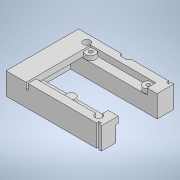
# Autodesk Inventor part: Стойка под электроннику
Saved by Autodesk Inventor 2020 (Build 240168000, 168)
## iProperties
Created: 2021-04-05
Part Number: Стойка под электроннику
Material: Типовые
Document SubType Name: Обычные детали
Designer: Антон
Density: 1 g/cm^3
Appearance: По умолчанию
Author: Антон
Autodesk Inventor part; units mm, degrees
ref_plane "YZ Plane" through (0, 0, 0) normal (1, 0, 0) x (0, 1, 0)
ref_plane "XZ Plane" through (0, 0, 0) normal (0, 1, 0) x (-1, 0, 0)
ref_plane "XY Plane" through (0, 0, 0) normal (0, 0, 1) x (1, 0, 0)
sketch "Эскиз1" plane through (0, 0, 0) normal (0, 1, 0) x (-1, 0, 0)
  line L0 (0, 0) -> (76, 0)
  line L1 (76, 0) -> (76, -57.8)
  line L2 (76, -57.8) -> (0, -57.8)
  line L3 (0, -57.8) -> (0, 0)
  line L4 (0, -28.9) -> (34.5, -28.9)
  line L5 (69, -13.4) -> (0, -13.4)
  line L6 (0, -13.4) -> (0, -44.4)
  line L7 (0, -44.4) -> (69, -44.4)
  line L8 (69, -44.4) -> (69, -13.4)
  line L9 (69, -13.4) -> (0, -44.4) construction
  line L10 (0, -13.4) -> (69, -44.4) construction
  line L11 (0, -13.4) -> (4, -13.4)
  point P0 (0, -13.4)
  dimension "d0" = 76
  dimension "d1" = 57.8
  dimension "d3" = 31
  dimension "d4" = 69
  constraints: 24 end point, 4 horizontal, 4 parallel, 3 midpoint, 2 perpendicular, 1 point on line
  measures "d0" distance of L1.end L2.end
  measures "d1" distance of L0.end L1.end
  measures "d3" distance of L6.end L5.end
  measures "d4" distance of L6.end L7.end
extrude "Выдавливание1" add sketch "Эскиз1" along normal blind 17.5 contours L0 L1 L2 L3 L7 L8 L5
sketch "Эскиз2" plane through (0, 17.5, 0) normal (0, 1, 0) x (1, 0, 0)
  line L0 (0, 0) -> (0, 6.4)
  line L1 (0, 0) -> (0, 57.8) projected
  line L2 (0, 6.4) -> (-8, 6.4)
  line L3 (-8, 6.4) -> (-60, 6.4)
  line L4 (-60, 6.4) -> (-60, 51.4)
  line L5 (-60, 51.4) -> (-8, 51.4)
  line L6 (-8, 51.4) -> (-8, 6.4)
  line L7 (-76, 57.8) -> (-76, 0) projected
  line L8 (-76, 0) -> (0, 0) projected
  point P0 (-60, 22)
  dimension "d9" = 6.4
  dimension "d10" = 8
  dimension "d11" = 52
  dimension "d12" = 45
  dimension "d16" = 57.8
  dimension "d17" = 76
  constraints: 12 end point, 2 parallel, 2 perpendicular, 2 point on line, 1 horizontal
  measures "d9" distance of L0.start L0.end
  measures "d10" distance of L0.end L2.end
  measures "d11" distance of L4.end L5.end
  measures "d12" distance of L3.end L4.end
  measures "d16" distance of L7.start L7.end
  measures "d17" distance of L7.end L0.start
extrude "Выдавливание2" cut sketch "Эскиз2" against normal blind 5
sketch "Эскиз29" plane through (-69, 0, -13.4) normal (1, 0, 0) x (0, 0, -1)
  line L0 (0, 17.5) -> (0, 12.5) projected
  line L1 (31, 12.5) -> (31, 17.5) projected
  line L2 (0, 17.5) -> (31, 17.5) projected
  line L3 (0, 12.5) -> (31, 12.5)
  point P0 (-13.4, 0)
  constraints: 2 end point, 1 perpendicular
extrude "Выдавливание23" add sketch "Эскиз29" along normal up to surface (9 mm away)
sketch "Эскиз3" plane through (0, 12.5, 0) normal (0, 1, 0) x (1, 0, 0)
  line L0 (-8, 6.4) -> (-60, 6.4) projected
  line L1 (-8, 51.4) -> (-8, 6.4) projected
  line L2 (-8, 51.4) -> (-11, 51.4)
  line L3 (-60, 51.4) -> (-8, 51.4) projected
  line L4 (-11, 51.4) -> (-11, 48.4)
  circle A0 centre (-11, 48.4) radius 4
  line L5 (-8, 6.4) -> (-60, 6.4) projected
  line L6 (-60, 51.4) -> (-8, 51.4) projected
  line L7 (-60, 51.4) -> (-57, 51.4)
  line L8 (-57, 51.4) -> (-57, 48.4)
  circle A1 centre (-57, 48.4) radius 4
  line L9 (-34, 6.4) -> (-34, 9.9)
  circle A2 centre (-34, 9.9) radius 3.5
  point P0 (-74.9, 17.65)
  point P1 (-74.9, 50.35)
  point P2 (-8, 44.4)
  point P3 (-8.3542, 51.4)
  point P4 (-8, 51.0458)
  point P5 (-59.6458, 51.4)
  point P6 (-54.3542, 51.4)
  dimension "d35" = 3
  dimension "d36" = 3
  dimension "d37" = 8
  dimension "d205" = 3
  dimension "d206" = 3
  dimension "d207" = 8
  dimension "d214" = 3.5
  dimension "d215" = 7
  constraints: 10 end point, 3 centre point, 3 coincident, 2 point on line, 2 vertical, 1 midpoint, 1 perpendicular
  measures "d35" distance of L1.start L2.end
  measures "d36" distance of L2.end L4.end
  measures "d37" diameter of A0
  measures "d205" distance of L3.start L7.end
  measures "d206" distance of L7.end L8.end
  measures "d207" diameter of A1
  measures "d214" distance of L9.start L9.end
  measures "d215" diameter of A2
extrude "Выдавливание5" add sketch "Эскиз3" along normal blind 3.5 contours L1 A0 L2 | A0 L1 | L1 A0 L3 L2 | L2 L3 A0 | L3 A1 | A2 picked at (-57.1322, 46.7573)
sketch "Эскиз4" plane through (-71.3, 16, -19.65) normal (0, 1, 0) x (0, 0, -1)
  arc A0 (31.75, -57.6542) -> (26.1042, -63.3) centre (28.75, -60.3) ccw projected
  line L0 (26.1042, -11.3) -> (31.3958, -11.3) projected
  arc A1 (26.1042, -11.3) -> (31.75, -16.9458) centre (28.75, -14.3) ccw projected
  line L1 (31.75, -11.6542) -> (31.75, -16.9458) projected
  arc A2 (31.75, -11.6542) -> (31.3958, -11.3) centre (28.75, -14.3) ccw projected
  point P0 (31.75, -57.1028)
  constraints: 2 coincident
hole "Отверстие1" at (-11, 16, -48.4) at (-57, 16, -48.4) direction (0, -1, 0) diameter 3 depth 5
sketch "Эскиз5" plane through (0, 12.5, 0) normal (0, 1, 0) x (1, 0, 0)
  line L0 (-60, 51.4) -> (-8, 51.4) projected
  line L1 (-8, 6.4) -> (-8.2, 6.4)
  line L2 (-8.2, 6.4) -> (-8.2, 6.05)
  line L3 (-8, 6.4) -> (-60, 6.4) projected
  line L4 (-60, 51.4) -> (-63.4, 51.4)
  line L5 (-63.4, 51.4) -> (-63.4, 51.75)
  line L6 (-8, 51.4) -> (-8, 6.4) projected
  point P0 (-21.2, 2.05)
  point P1 (-57.2, 6.4)
  point P2 (-8, 44.4)
  point P3 (-20.7569, 6.4)
  point P4 (-60, 6.4)
  dimension "d196" = 0.35
  dimension "d200" = 0.35
  dimension "d208" = 3.4
  dimension "d209" = 0.2
  constraints: 8 end point, 2 perpendicular, 1 horizontal, 1 point on line, 1 other
  measures "d196" distance of L4.end L5.end
  measures "d200" distance of L1.end L2.end
  measures "d208" distance of L0.start L4.end
  measures "d209" distance of L1.start L1.end
hole "Отверстие2" at (-63.4, 12.5, -51.75) at (-8.2, 12.5, -6.05) direction (0, -1, 0) diameter 3.2 end through all countersink diameter 5.8 countersink angle 90
sketch "Эскиз27" plane through (0, 12.5, 0) normal (0, 1, 0) x (1, 0, 0)
  arc A0 (-53.0282, 48.8739) -> (-50.5212, 51.4) centre (-53.4, 51.75) ccw projected
  circle A1 centre (-63.4, 51.75) radius 2.9 projected
  circle A2 centre (-63.4, 51.75) radius 1.6 projected
  circle A3 centre (-8.2, 6.05) radius 1.6 projected
  arc A4 (-11.0788, 6.4) -> (-8, 8.9431) centre (-8.2, 6.05) ccw projected
  line L0 (-8, 8.9431) -> (-8, 6.4) projected
  line L1 (-8, 6.4) -> (-11.0788, 6.4) projected
  line L2 (-8, 6.4) -> (-60, 6.4) projected
  line L3 (-34, 6.4) -> (-34, 10.4)
  point P0 (0, 0)
  point P1 (-65, 49.3313)
  point P2 (-50.5212, 51.4)
  dimension "d213" = 4
  constraints: 2 end point, 1 midpoint, 1 vertical
  measures "d213" distance of L3.start L3.end
extrude "Выдавливание21" cut sketch "Эскиз27" along normal up to surface (5 mm away) contours A1 | A2 | A3 L1 L0 | A3 L0 A4 L1 picked at (-8.6134, 5.2227)
sketch "Эскиз10" plane through (0, 0, 0) normal (0, -1, 0) x (1, 0, 0)
  line L0 (0, 0) -> (0, -13.4) projected
  line L1 (0, -13.4) -> (-4, -13.4)
  line L2 (-4, -13.4) -> (-4, -11.4)
  line L3 (-4, -11.4) -> (0, -11.4)
  line L4 (0, -11.4) -> (0, -13.4)
  dimension "d109" = 4
  dimension "d110" = 2
  constraints: 8 end point, 2 parallel, 1 horizontal, 1 perpendicular
  measures "d109" distance of L2.end L3.end
  measures "d110" distance of L1.end L2.end
extrude "Выдавливание9" cut sketch "Эскиз10" against normal up to surface (12.5 mm away)
sketch "Эскиз11" plane through (-76, 0, 0) normal (0, 0, 1) x (1, 0, 0)
  line L0 (76, 0) -> (76, 17.5) projected
  line L1 (76, 0) -> (76, 0)
  line L2 (76, 17.5) -> (76, 17.5)
  line L3 (76, 0) -> (74, 0)
  line L4 (76, 17.5) -> (74, 17.5)
  line L5 (74, 0) -> (72, 0)
  line L6 (72, 0) -> (72, 17.5)
  line L7 (72, 17.5) -> (74, 17.5)
  line L8 (74, 17.5) -> (74, 0)
  line L9 (0, 17.5) -> (76, 17.5) projected
  dimension "d113" = 2
  dimension "d115" = 2
  constraints: 16 end point, 3 horizontal, 2 equal length, 2 parallel, 2 point on line, 1 collinear, 1 perpendicular
  measures "d113" distance of L1.end L3.end
  measures "d115" distance between parallel lines of L8 L6
extrude "Выдавливание10" cut sketch "Эскиз11" against normal blind 2 contours L5 L6 L7 L8
ref_plane "РабПлоскость2" through (-76, 0, -28.9) normal (0, 0, 1) x (1, 0, 0)
mirror "Зеркальное отражение1" about plane through (-76, 0, -28.9) normal (0, 0, 1) of "Выдавливание10"
sketch "Эскиз12" plane through (0, 0, 0) normal (0, -1, 0) x (1, 0, 0)
  line L0 (-36, -57.8) -> (-40, -57.8) construction
  line L1 (0, -57.8) -> (-76, -57.8) projected
  line L2 (-36, -55.75) -> (-40, -55.75)
  line L3 (-40, -59.85) -> (-36, -59.85)
  arc A0 (-36, -59.85) -> (-36, -55.75) centre (-36, -57.8) ccw
  arc A1 (-40, -55.75) -> (-40, -59.85) centre (-40, -57.8) ccw
  line L4 (-60, -51.4) -> (-60, -6.4) projected
  line L5 (-60, -51.4) -> (-8, -51.4) projected
  line L6 (-8, -51.4) -> (-8, -44.4) projected
  line L7 (-8, -44.4) -> (0, -44.4) projected
  line L8 (0, -44.4) -> (0, -57.8) projected
  line L9 (0, -57.8) -> (-2, -57.8) projected
  line L10 (-76, -57.8) -> (-76, 0) projected
  line L11 (-76, 0) -> (-4, 0) projected
  line L12 (0, 0) -> (0, -13.4) projected
  line L13 (0, -13.4) -> (-8, -13.4) projected
  line L14 (-8, -13.4) -> (-8, -8.9431) projected
  line L15 (-11.0788, -6.4) -> (-60, -6.4) projected
  line L16 (-36, -55.75) -> (-40, -55.75)
  line L17 (-2, -57.8) -> (-2, -55.8) projected
  line L18 (-2, -55.8) -> (-4, -55.8) projected
  line L19 (-4, -55.8) -> (-4, -57.8) projected
  line L20 (-4, -57.8) -> (-76, -57.8) projected
  line L21 (-4, 0) -> (-4, -2) projected
  line L22 (-4, -2) -> (-2, -2) projected
  line L23 (-2, -2) -> (-2, 0) projected
  line L24 (-2, 0) -> (0, 0) projected
  circle A2 centre (-63.4, -51.75) radius 2.9 projected
  arc A3 (-8, -8.9431) -> (-11.0788, -6.4) centre (-8.2, -6.05) ccw projected
  point P0 (-38, -57.8)
  point P1 (-41, -51.4)
  point P2 (-35, -51.4)
  point P3 (-42.05, -57.8)
  point P4 (-33.95, -57.8)
  point P5 (-35, -51.4)
  point P6 (-42.05, -57.8)
  point P7 (-33.95, -57.8)
  point P8 (-4, -57.8)
  point P9 (-2, -57.8)
  dimension "d118" = 2
  dimension "d210" = 2.05
  constraints: 10 end point, 4 point on circle, 4 tangent, 2 centre point, 2 midpoint, 1 horizontal, 1 parallel, 1 point on line
  measures "d118" distance of point (-38, -57.8) L0.end
  measures "d210" radius of A1
extrude "Выдавливание11" cut sketch "Эскиз12" against normal through all contours L1 L19 L18 L17 | A0 L3 A1 L1 | L1 A1 L2 A0
sketch "Эскиз14" plane through (0, 17.5, 0) normal (0, 1, 0) x (1, 0, 0)
  line L0 (-60, 51.4) -> (-8, 51.4) projected
  line L1 (-38, 51.4) -> (-38, 53.0067)
  line L2 (0, 57.8) -> (-2, 57.8) projected
  line L3 (-32.95, 57.8) -> (-30.95, 57.8)
  line L4 (-30.95, 57.8) -> (-30.95, 49.4)
  line L5 (-30.95, 49.4) -> (-32.95, 49.4)
  line L6 (-32.95, 49.4) -> (-32.95, 57.8)
  line L7 (-30.95, 49.4) -> (-45.05, 49.4)
  line L8 (-45.05, 49.4) -> (-45.05, 51.4)
  line L9 (-45.05, 51.4) -> (-30.95, 51.4)
  line L10 (-30.95, 51.4) -> (-30.95, 49.4)
  line L11 (-45.05, 49.4) -> (-43.05, 49.4)
  line L12 (-43.05, 49.4) -> (-43.05, 57.8)
  line L13 (-43.05, 57.8) -> (-45.05, 57.8)
  line L14 (-45.05, 57.8) -> (-45.05, 49.4)
  line L15 (-60, 51.4) -> (-8, 51.4) projected
  line L16 (-40, 55.75) -> (-36, 55.75) projected
  line L17 (-41, 51.4) -> (-34.5, 51.4) projected
  line L18 (-36, 55.75) -> (-40, 55.75) projected
  line L19 (-4, 57.8) -> (-33.95, 57.8) projected
  line L20 (-42.05, 57.8) -> (-76, 57.8) projected
  point P0 (0, 0)
  point P1 (-28.95, 57.8)
  point P2 (-32.95, 51.4)
  point P3 (-47.05, 54.4893)
  point P4 (-49.4, 51.4)
  point P5 (-43.05, 51.4)
  point P6 (-34.5, 51.4)
  point P7 (-30.95, 51.4)
  point P8 (-34.5, 51.4)
  point P9 (-38, 55.75)
  dimension "d136" = 2
  dimension "d137" = 2
  dimension "d211" = 1
  dimension "d212" = 1
  constraints: 26 end point, 6 parallel, 4 collinear, 3 horizontal, 3 perpendicular, 2 midpoint, 2 point on line, 1 vertical, 1 other
  measures "d136" distance between parallel lines of L6 L4
  measures "d137" distance between parallel lines of L9 L7
  measures "d211" distance from line of L6 L19.end
  measures "d212" distance from line of L12 L20.start
ref_plane "РабПлоскость4" through (0, 8.75, 0) normal (0, 1, 0) x (1, 0, 0)
extrude "Выдавливание12" cut sketch "Эскиз14" against normal mid plane 5 from surface at -8.75
chamfer "Фаска5" distance 1 angle 45 4 edges at (-32.95, 8.75, -51.4) (-43.05, 8.75, -51.4) (-45.05, 8.75, -49.4) (-30.95, 8.75, -49.4)
sketch "Эскиз21" plane through (0, 0, 0) normal (0, -1, 0) x (1, 0, 0)
  line L0 (-74, -2.7) -> (-49, -2.7)
  line L1 (-49, -2.7) -> (-49, -10.7)
  line L2 (-49, -10.7) -> (-74, -10.7)
  line L3 (-74, -10.7) -> (-74, -2.7)
  line L4 (-76, 0) -> (-4, 0) projected
  line L5 (-76, -57.8) -> (-76, 0) projected
  point P0 (0, 0)
  dimension "d167" = 8
  dimension "d168" = 25
  dimension "d169" = 2.7
  dimension "d170" = 2
  constraints: 8 end point, 2 parallel, 1 horizontal, 1 perpendicular
  measures "d167" distance of L0.end L1.end
  measures "d168" distance of L1.end L2.end
  measures "d169" distance between parallel lines of L4 L0
  measures "d170" distance between parallel lines of L5 L3
extrude "Выдавливание17" cut sketch "Эскиз21" against normal blind 13.5
sketch "Эскиз22" plane through (-76, 0, -57.8) normal (-1, 0, 0) x (0, 0, 1)
  line L0 (47.1, 0) -> (55.1, 0) projected
  line L1 (47.1, 0) -> (47.1, 13.5) projected
  line L2 (47.1, 13.5) -> (55.1, 13.5) projected
  line L3 (55.1, 0) -> (55.1, 13.5) projected
  line L4 (47.1, 0) -> (47.1, 13.5) projected
  line L5 (47.1, 6.75) -> (55.1, 6.75)
  point P0 (57.8, 0)
  point P1 (51.1, 6.75)
  constraints: 3 midpoint, 2 end point
hole "Отверстие4" at (-76, 6.75, -6.7) direction (1, 0, 0) diameter 6.5 depth 2
sketch "Эскиз25" plane through (0, 17.5, 0) normal (0, 1, 0) x (1, 0, 0)
  line L0 (-76, 0) -> (-4, 0) projected
  line L1 (-60, 6.4) -> (-60, 10.7) projected
  line L2 (-60, 6.4) -> (-58.5, 6.4)
  line L3 (-58.5, 6.4) -> (-58.5, 0)
  line L4 (-58.5, 0) -> (-60, 0)
  line L5 (-60, 0) -> (-60, 6.4)
  line L6 (-76, 0) -> (-4, 0) projected
  point P0 (0, 0)
  point P1 (-60, 0)
  point P2 (-58.5, 0)
  dimension "d195" = 1.5
  constraints: 8 end point, 2 parallel, 1 collinear, 1 horizontal, 1 perpendicular
  measures "d195" distance of L3.end L4.end
extrude "Выдавливание19" cut sketch "Эскиз25" against normal up to surface (5 mm away)
sketch "Эскиз30" plane through (0, 0, 0) normal (0, -1, 0) x (1, 0, 0)
  line L0 (-76, -44) -> (-74, -44)
  line L1 (-74, -44) -> (-74, -13.8)
  line L2 (-74, -13.8) -> (-76, -13.8)
  line L3 (-76, -13.8) -> (-76, -44)
  line L4 (-76, -57.8) -> (-76, 0) projected
  line L5 (-74, -44) -> (-75.1, -44)
  line L6 (-75.1, -44) -> (-75.1, -45)
  line L7 (-75.1, -45) -> (-74, -45)
  line L8 (-74, -45) -> (-74, -44)
  line L9 (-74, -13.8) -> (-75.5, -13.8)
  line L10 (-75.5, -13.8) -> (-75.5, -12.8)
  line L11 (-75.5, -12.8) -> (-74, -12.8)
  line L12 (-74, -12.8) -> (-74, -13.8)
  point P0 (0, 0)
  point P1 (-76, -28.9)
  point P2 (-75.5, -13.8)
  dimension "d216" = 30.2
  dimension "d217" = 2
  dimension "d218" = 1.1
  dimension "d219" = 1
  dimension "d220" = 1.5
  dimension "d221" = 1
  constraints: 24 end point, 6 parallel, 3 horizontal, 3 perpendicular, 2 midpoint
  measures "d216" distance of L0.end L1.end
  measures "d217" distance of L0.start L0.end
  measures "d218" distance of L7.end L6.end
  measures "d219" distance of L7.end L0.end
  measures "d220" distance of L10.end L11.end
  measures "d221" distance of L9.end L10.end
extrude "Выдавливание24" cut sketch "Эскиз30" against normal blind 15.15
equation "\"d9\" = -0.5 * d12 + 0.5 * d16"
